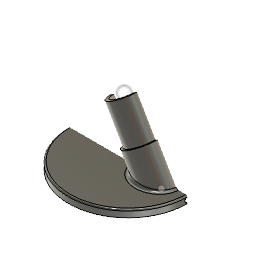
base-plate-simple-cable-hole (Autodesk Fusion 360 design; units mm, degrees)
Autodesk Fusion 360 part; units mm, degrees
sketch "Skizze1" plane through (0, 0, 0) normal (0, 0, 1) x (1, 0, 0)
  circle A0 centre (0, 0) radius 80
extrude "Extrusion1" add sketch "Skizze1" along normal blind 10 makes body 1
fillet "Abrundung1" radius 2 1 edges at (-74.5862, -28.9292, 10) on bodies 1
sketch "Skizze2" plane through (0, 0, 0) normal (0, 1, 0) x (1, 0, 0)
  line L0 (45, 0) -> (-5, -86.6025) construction
ref_plane "Arbeitsebene1" through (-5, 0, 86.6025) normal (-0.5, 0, 0.866025) x (0, -1, 0)
sketch "Skizze3" plane through (-5, 0, 86.6025) normal (-0.5, 0, 0.866025) x (0, -1, 0)
  circle A0 centre (0, 0) radius 23
  circle A1 centre (0, 0) radius 20
extrude "Extrusion5" add sketch "Skizze3" against normal blind 110 separate body contours A0 | A1 makes body 2
combine "Kombinieren1" operation add target body 1 tool bodies 2
extrude "Extrusion6" cut sketch "Skizze3" against normal blind 50 bodies 1
fillet "Abrundung2" radius 4 3 edges at (65.7846, 0, 10) (-74.5862, -28.9292, 8) (-72.7215, 28.206, 10) on bodies 1
sketch "Skizze4" plane through (-5, 0, 86.6025) normal (-0.5, 0, 0.866025) x (0, -1, 0)
  circle A0 centre (0, 0) radius 15.75
extrude "Extrusion7" cut sketch "Skizze4" against normal blind 110 bodies 1
sketch "Skizze5" plane through (0, 0, 0) normal (0, 0, 1) x (1, 0, 0)
  circle A0 centre (0, 0) radius 160
extrude "Extrusion8" cut sketch "Skizze5" against normal blind 110 bodies 1
ref_plane "Arbeitsebene2" through (70, 0, 0) normal (1, 0, 0) x (0, 1, 0)
sketch "Skizze6" plane through (70, 0, 0) normal (1, 0, 0) x (0, 0, -1)
  circle A0 centre (-4.5, 0) radius 3
extrude "Extrusion9" cut sketch "Skizze6" along normal mid plane 32 bodies 1
chamfer "Fase1" distance 0.3 angle 45 2 edges at (60.3709, 2.9933, 4.3029) (79.9437, -3, 4.5) on bodies 1
equation "base_plate_diameter = 160 mm" comment "Durchmesser der runden Basis-Platte"
equation "base_plate_height = 10 mm" comment "Höhe der runden Basis-Platte"
equation "base_plate_rounding = 2 mm" comment "Abrundung der oberen Basis-Platte-Kante (Kreis)"
equation "leg_outer_diameter = 46 mm" comment "Aussendurchmesser der Röhre"
equation "ring_inner_diameter = 40 mm" comment "Aussendurchmesser des oberen Röhrensegments (Stufenabsatz)"
equation "ring_extrude_depth = 50 mm" comment "Länge des oberen (dünnen) Röhrensegments / Stufenabsatz"
equation "hole_inner_diameter = 31.5 mm" comment "Innendurchmesser der Röhre (Loch)"
equation "leg_length = 100 mm" comment "Laenge der Röhre"
equation "leg_angle = 120 deg" comment "Winkel des Beines zur XY-Ebene (Innenwinkel an der Platte)"
equation "leg_offset = 45 mm" comment "Abstand des Bein-Fußpunktes vom Plattenmittelpunkt"
equation "leg_plate_rounding = 4 mm" comment "Abrundung der Kante: Bein und Platte (wird bei Solver-Problemen automatisch verkleinert)"
equation "cable_hole_offset = 70 mm" comment "Versatz der Kabelkanal-Konstruktionsebene zur YZ-Ebene"
equation "cable_hole_diameter = 6 mm" comment "Durchmesser des Kabelkanallochs"
equation "cable_hole_height = 4.5 mm" comment "Höhe des Kabelkanallochs über der Unterseite (8.0mm)"
equation "cable_hole_chamfer = 0.3 mm" comment "Abfasung der Lochkanten des Kabelkanals"
equation "d16 = base_plate_height"
equation "d19 = base_plate_rounding"
equation "d27 = -( leg_length + base_plate_height )"
equation "d29 = -ring_extrude_depth"
equation "d32 = leg_plate_rounding"
equation "d33 = -leg_length - base_plate_height"
equation "d35 = -( leg_length + base_plate_height )"
equation "d41 = cable_hole_chamfer"
